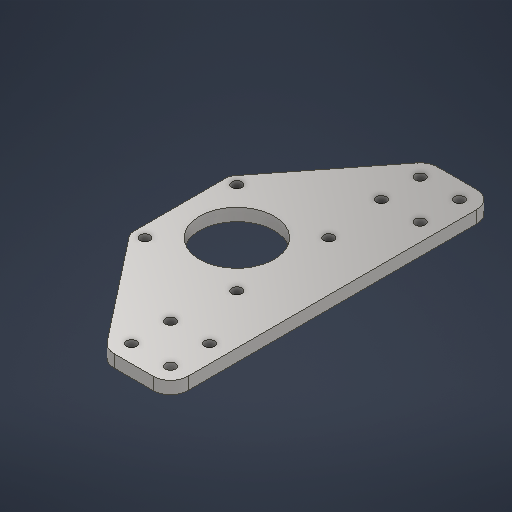
# Autodesk Inventor part: CNC-000-StructureGusset1
Saved by Autodesk Inventor 2026.2 (Build 302298000, 298)
## iProperties
Created: 2026-06-14
Part Number: CNC-000-StructureGusset1
Material: Steel AISI 1008 91 HR
Document SubType Name: Modeling
Designer: Kenji
Density: 7.872 g/cm^3
Appearance: Steel
Mass: 447.876 g
Surface Area: 225.974 cm^2
Volume: 56.8948 cm^3
Author: Kenji
Autodesk Inventor part; units mm, degrees
ref_plane "YZ Plane" through (0, 0, 0) normal (1, 0, 0) x (0, 1, 0)
ref_plane "XZ Plane" through (0, 0, 0) normal (0, 1, 0) x (-1, 0, 0)
ref_plane "XY Plane" through (0, 0, 0) normal (0, 0, 1) x (1, 0, 0)
sketch "Sketch1" plane through (0, 0, 0) normal (0, 1, 0) x (-1, 0, 0)
  circle A0 centre (0, 0) radius 2.6
  line L0 (0, 0) -> (0, -2.6) construction
  line L1 (0, 0) -> (-2.6, 0) construction
  circle A1 centre (0, -20) radius 2.6
  circle A2 centre (-20, 0) radius 2.6
  circle A3 centre (-20, -20) radius 2.6
  circle A4 centre (0, 108) radius 2.6
  circle A5 centre (-20, 108) radius 2.6
  circle A6 centre (0, 128) radius 2.6
  circle A7 centre (-20, 128) radius 2.6
  circle A8 centre (20, 54) radius 19.15
  circle A9 centre (43.57, 30.43) radius 2.6
  circle A10 centre (-3.57, 30.43) radius 2.6
  circle A11 centre (-3.57, 77.57) radius 2.6
  circle A12 centre (43.57, 77.57) radius 2.6
  circle A13 centre (43.57, 77.57) radius 5.775 construction
  circle A14 centre (43.57, 30.43) radius 5.775 construction
  circle A15 centre (0, 128) radius 8.95 construction
  circle A16 centre (-20, 128) radius 8.95 construction
  circle A17 centre (0, -20) radius 8.95 construction
  circle A18 centre (-20, -20) radius 8.95 construction
  line L2 (7.0435, 133.5219) -> (48.1148, 81.133)
  line L3 (48.1148, 26.867) -> (7.0435, -25.5219)
  line L4 (0, 136.95) -> (-20, 136.95)
  line L5 (-28.95, 128) -> (-28.95, -20)
  line L6 (-20, -28.95) -> (0, -28.95)
  line L7 (49.345, 77.57) -> (49.345, 30.43)
  arc A19 (49.345, 77.57) -> (48.1148, 81.133) centre (43.57, 77.57) ccw
  arc A20 (48.1148, 26.867) -> (49.345, 30.43) centre (43.57, 30.43) ccw
  arc A21 (0, -28.95) -> (7.0435, -25.5219) centre (0, -20) ccw
  arc A22 (-28.95, -20) -> (-20, -28.95) centre (-20, -20) ccw
  arc A23 (-20, 136.95) -> (-28.95, 128) centre (-20, 128) ccw
  arc A24 (7.0435, 133.5219) -> (0, 136.95) centre (0, 128) ccw
  point P0 (0, -22.6)
  point P1 (-2.6, -20)
  point P2 (-20, -2.6)
  point P3 (-22.6, 0)
  point P4 (-20, -22.6)
  point P5 (-22.6, -20)
  dimension "d0" = 5.2
  dimension "d3" = 20
  dimension "d6" = 20
  dimension "d9" = 108
  dimension "d10" = 20
  dimension "d11" = 20
  dimension "d13" = 54
  dimension "d14" = 38.3
  dimension "d15" = 23.57
  dimension "d16" = 23.57
  dimension "d17" = 47.14
  dimension "d18" = 47.14
  dimension "d19" = 3.175
  dimension "d20" = 6.35
  constraints: 32 point on circle, 25 centre point, 16 end point, 16 equal radius, 12 tangent, 6 vertical alignment, 5 coincident, 4 horizontal alignment, 3 perpendicular, 2 horizontal, 2 vertical, 1 concentric, 12 other
  measures "d0" diameter of A0
  measures "d3" distance of L0.start A1.centre
  measures "d6" distance of L0.start A2.centre
  measures "d9" distance of point (0, 0) A4.centre
  measures "d10" distance of A6.centre A4.centre
  measures "d11" horizontal distance of point (0, 0) A8.centre
  measures "d13" vertical distance of A8.centre point (0, 0)
  measures "d14" diameter of A8
  measures "d15" horizontal distance of A9.centre A8.centre
  measures "d16" horizontal distance of A8.centre A9.centre
  measures "d17" distance of A11.centre A12.centre
  measures "d18" distance of A9.centre A12.centre
  measures "d19" radial gap between concentric circles of A12 A13
  measures "d20" radial gap between concentric circles of A15 A6
extrude "Extrusion1" add sketch "Sketch1" along normal blind 6.35
equation "\"d13\" = 0.5 * d9"
equation "\"d18\" = d17"
body "Solid1"
